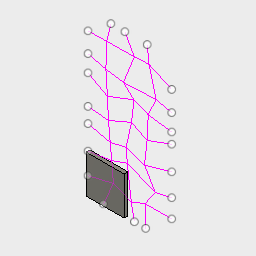
Untitled (Autodesk Fusion 360 design; units mm, degrees)
Autodesk Fusion 360 part; units mm, degrees
sketch "Sketch1" plane through (0, 0, 0) normal (0, 0, 1) x (1, 0, 0)
  line L0 (0, 0) -> (100, 0)
  line L1 (100, 0) -> (100, 100.1527)
  line L2 (100, 100.1527) -> (0, 100.1527)
  line L3 (0, 100.1527) -> (0, 0)
  dimension "d1" = 100
  constraint horizontal L0
  constraint vertical L1
  constraint horizontal L2
  constraint vertical L3
  constraint coincident L0.start L3.end
extrude "Extrude1" add sketch "Sketch1" along normal blind 10
sketch "Mesh (Cut)" plane through (0, 0, 0) normal (0, 0, 1) x (1, 0, 0)
  line L0 (-5, 39.0427) -> (61.6007, 54.6023)
  line L1 (61.6007, 54.6023) -> (108.5344, 36.1486)
  line L2 (108.5344, 36.1486) -> (144.7267, 50.0901)
  line L3 (144.7267, 50.0901) -> (215, 50.6439)
  line L4 (215, 98.8135) -> (171.6674, 89.0622)
  line L5 (171.6674, 89.0622) -> (98.1932, 118.8908)
  line L6 (98.1932, 118.8908) -> (57.4917, 104.6282)
  line L7 (57.4917, 104.6282) -> (-5, 95.0002)
  line L8 (-5, 157.4229) -> (53.1384, 143.8198)
  line L9 (53.1384, 143.8198) -> (95.0995, 153.6126)
  line L10 (95.0995, 153.6126) -> (143.3819, 137.4587)
  line L11 (143.3819, 137.4587) -> (215, 157.6864)
  line L12 (215, 220.6611) -> (150.0272, 196.6581)
  line L13 (150.0272, 196.6581) -> (109.1269, 217.3192)
  line L14 (109.1269, 217.3192) -> (48.7593, 191.5312)
  line L15 (48.7593, 191.5312) -> (-5, 196.7083)
  line L16 (-5, 272.9227) -> (45.849, 245.1239)
  line L17 (45.849, 245.1239) -> (115.9062, 271.9292)
  line L18 (115.9062, 271.9292) -> (153.246, 256.6474)
  line L19 (153.246, 256.6474) -> (215, 248.4268)
  line L20 (215, 292.3366) -> (173.7576, 301.7205)
  line L21 (173.7576, 301.7205) -> (87.9856, 297.7158)
  line L22 (87.9856, 297.7158) -> (41.9186, 304.7838)
  line L23 (41.9186, 304.7838) -> (-5, 316.6761)
  line L24 (-5, 368.5301) -> (43.8508, 369.3265)
  line L25 (43.8508, 369.3265) -> (116.7114, 370.3208)
  line L26 (116.7114, 370.3208) -> (155.0718, 372.5459)
  line L27 (155.0718, 372.5459) -> (215, 345.2945)
  line L28 (35.5536, -5) -> (61.6007, 54.6023)
  line L29 (61.6007, 54.6023) -> (57.4917, 104.6282)
  line L30 (57.4917, 104.6282) -> (53.1384, 143.8198)
  line L31 (53.1384, 143.8198) -> (48.7593, 191.5312)
  line L32 (48.7593, 191.5312) -> (45.849, 245.1239)
  line L33 (45.849, 245.1239) -> (41.9186, 304.7838)
  line L34 (41.9186, 304.7838) -> (43.8508, 369.3265)
  line L35 (43.8508, 369.3265) -> (55.2024, 415)
  line L36 (91.9506, 415) -> (116.7114, 370.3208)
  line L37 (116.7114, 370.3208) -> (87.9856, 297.7158)
  line L38 (87.9856, 297.7158) -> (115.9062, 271.9292)
  line L39 (115.9062, 271.9292) -> (109.1269, 217.3192)
  line L40 (109.1269, 217.3192) -> (95.0995, 153.6126)
  line L41 (95.0995, 153.6126) -> (98.1932, 118.8908)
  line L42 (98.1932, 118.8908) -> (108.5344, 36.1486)
  line L43 (108.5344, 36.1486) -> (116.8599, -5)
  line L44 (146.67, -5) -> (144.7267, 50.0901)
  line L45 (144.7267, 50.0901) -> (171.6674, 89.0622)
  line L46 (171.6674, 89.0622) -> (143.3819, 137.4587)
  line L47 (143.3819, 137.4587) -> (150.0272, 196.6581)
  line L48 (150.0272, 196.6581) -> (153.246, 256.6474)
  line L49 (153.246, 256.6474) -> (173.7576, 301.7205)
  line L50 (173.7576, 301.7205) -> (155.0718, 372.5459)
  line L51 (155.0718, 372.5459) -> (150.4899, 415)
